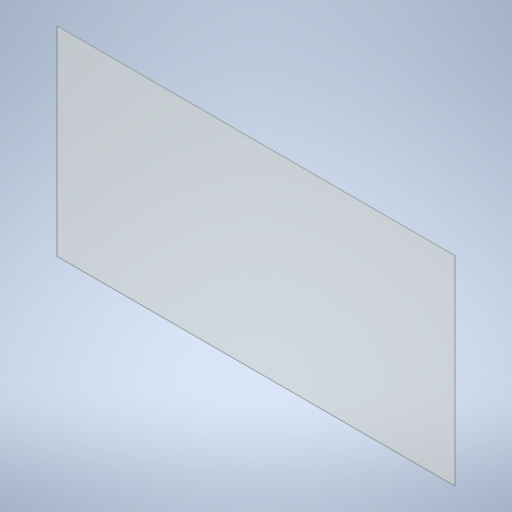
# Autodesk Inventor part: Clear Panel
Saved by Autodesk Inventor 2024 (Build 280153000, 153)
## iProperties
Created: 2024-02-22
Part Number: Clear Panel
Material: Generic
Document SubType Name: Modeling
Designer: flynf
Density: 1 g/cm^3
Appearance: Clear
Author: flynf
Autodesk Inventor part; units mm, degrees
ref_plane "YZ Plane" through (0, 0, 0) normal (1, 0, 0) x (0, 1, 0)
ref_plane "XZ Plane" through (0, 0, 0) normal (0, 1, 0) x (-1, 0, 0)
ref_plane "XY Plane" through (0, 0, 0) normal (0, 0, 1) x (1, 0, 0)
sketch "Sketch1" plane through (0, 0, 0) normal (0, 0, 1) x (1, 0, 0)
  line L0 (0, 0) -> (2038.35, 0)
  line L1 (2038.35, 0) -> (2038.35, 1022.35)
  line L2 (2038.35, 1022.35) -> (0, 1022.35)
  line L3 (0, 1022.35) -> (0, 0)
  dimension "d0" = 2038.35
  dimension "d1" = 1022.35
  constraints: 8 end point, 2 parallel, 1 horizontal, 1 perpendicular
  measures "d0" distance of L2.end L1.end
  measures "d1" distance of L1.end L0.end
extrude "Extrusion1" add sketch "Sketch1" along normal blind 3.175
body "Solid1"
